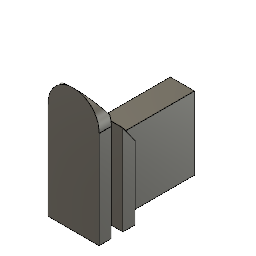
1010RailButton (Autodesk Fusion 360 design; units mm, degrees)
Autodesk Fusion 360 part; units mm, degrees
note: some values were not read from the file. Set by a fixed rule: which sketch regions a step uses.
sketch "Sketch1" plane through (0, 0, 0) normal (0, 0, 1) x (1, 0, 0)
  circle A0 centre (0, 0) radius 5.25
  dimension "d1" = 10.5
  constraint coincident A0.centre origin
  measures "d1" diameter of A0
extrude "Extrude1" add sketch "Sketch1" along normal blind 2.5 makes body 1
sketch "Sketch2" plane through (0, 0, 2.5) normal (0, 0, 1) x (1, 0, 0)
  circle A0 centre (0, 0) radius 5.25
  circle A1 centre (0, 0) radius 2.75
  dimension "d4" = 5.5
  constraint concentric A0 A1
  measures "d4" diameter of A1
extrude "Extrude2" add sketch "Sketch2" along normal blind 2.4 contours A1 bodies 1
sketch "Sketch3" plane through (0, 0, 4.9) normal (0, 0, 1) x (1, 0, 0)
  circle A0 centre (0, 0) radius 2.75
  circle A1 centre (0, 0) radius 5.25
  dimension "d7" = 10.5
  constraint concentric A0 A1
  measures "d7" diameter of A1
extrude "Extrude3" add sketch "Sketch3" along normal blind 2.5 contours A0 | A1 bodies 1
fillet "Fillet1" radius 0.5 2 edges at (-2.5639, 0.9944, 2.5) (-2.5639, -0.9944, 4.9) on bodies 1
sketch "Sketch4" plane through (0, 0, 0) normal (0, 0, -1) x (-1, 0, 0)
  circle A0 centre (0, 0) radius 5.25
  circle A1 centre (0, 0) radius 2.75
  dimension "d11" = 5.5
  constraint concentric A0 A1
  measures "d11" diameter of A1
extrude "Extrude4" add sketch "Sketch4" along normal blind 10 contours A1 bodies 1
fillet "Fillet2" radius 0.5 1 edges at (2.5639, 0.9944, 0) on bodies 1
delete_body "RemoveBody1" bodies 1
sketch "Sketch5" plane through (0, 0, 0) normal (0, 1, 0) x (1, 0, 0)
sketch "Sketch6" plane through (0, 0, 0) normal (0, 0, 1) x (1, 0, 0)
  line L0 (0, 0) -> (5.25, 0)
  line L1 (0, 0) -> (-5.25, 0)
  line L2 (5.25, 0) -> (5.25, 15)
  line L3 (5.25, 15) -> (-5.25, 15)
  line L4 (-5.25, 15) -> (-5.25, 0)
  circle A0 centre (0, 15) radius 5.25
  dimension "d15" = 5.25
  dimension "d16" = 5.25
  dimension "d17" = 15
  dimension "d18" = 10.5
  constraint coincident L0.start L1.start
  constraint horizontal L0
  constraint parallel L0 L1
  constraint perpendicular L0 L2
  constraint perpendicular L2 L3
  constraint perpendicular L1 L4
  constraint midpoint L3 A0.centre
  measures "d15" distance of L0.start L0.end
  measures "d16" distance of L0.start L1.end
  measures "d17" distance of L0.end L2.end
  measures "d18" diameter of A0
extrude "Extrude5" add sketch "Sketch6" along normal blind 2.5 separate body makes body 2
sketch "Sketch7" plane through (0, 0, 2.5) normal (0, 0, 1) x (1, 0, 0)
  line L0 (-5.25, 0) -> (5.25, 0)
  line L1 (5.25, 0) -> (5.25, 15)
  arc A0 (5.25, 15) -> (-5.25, 15) centre (0, 15) ccw
  line L2 (-5.25, 15) -> (-5.25, 0)
  line L3 (0, 0) -> (2.75, 0)
  line L4 (0, 0) -> (-2.75, 0)
  line L5 (-2.75, 0) -> (-2.75, 12.5)
  line L6 (2.75, 0) -> (2.75, 12.5)
  line L7 (2.75, 12.5) -> (-2.75, 12.5)
  circle A1 centre (0, 12.5) radius 2.75
  dimension "d21" = 2.75
  dimension "d22" = 2.75
  dimension "d23" = 12.5
  dimension "d24" = 5.5
  constraint coincident L3.start L4.start
  constraint coincident L0 L3.end
  constraint parallel L0 L4
  constraint perpendicular L0 L5
  constraint perpendicular L0 L6
  constraint perpendicular L5 L7
  constraint midpoint L7 A1.centre
  measures "d21" distance of L3.start L3.end
  measures "d22" distance of L3.start L4.end
  measures "d23" distance of L4.end L5.end
  measures "d24" diameter of A1
extrude "Extrude6" add sketch "Sketch7" along normal blind 2.4 contours L0 L3 L4 L5 L6 A1 | L7 A1 | L7 A1 bodies 2
sketch "Sketch8" plane through (0, 0, 4.9) normal (0, 0, 1) x (1, 0, 0)
  line L0 (-2.75, 0) -> (2.75, 0)
  line L1 (2.75, 0) -> (2.75, 12.5)
  arc A0 (2.75, 12.5) -> (-2.75, 12.5) centre (0, 12.5) ccw
  line L2 (-2.75, 12.5) -> (-2.75, 0)
  circle A1 centre (0, 15.25) radius 5.25
  line L3 (0, 0) -> (5.25, 0)
  line L4 (5.25, 0) -> (5.25, 15)
  line L5 (0, 0) -> (-5.25, 0)
  line L6 (-5.25, 0) -> (-5.25, 15.25)
  line L7 (5.25, 15) -> (-5.25, 15)
  dimension "d27" = 10.5
  dimension "d39" = 5.25
  dimension "d40" = 15
  dimension "d41" = 5.25
  dimension "d42" = 10.5
  constraint midpoint A0 A1.centre
  constraint coincident L3.start L5.start
  constraint parallel L0 L3
  constraint perpendicular L3 L4
  constraint perpendicular L4 L5
  constraint coincident A1 L6.end
  constraint tangent A1 L6
  constraint perpendicular L4 L7
  measures "d27" diameter of A1
  measures "d39" distance of L3.start L3.end
  measures "d40" distance of L3.end L4.end
  measures "d41" distance of L3.start L5.end
  measures "d42" distance of L4.end L7.end
extrude "Extrude10" add sketch "Sketch8" along normal blind 2.5 contours L0 L1 L2 A1 L3 L5 | L2 A1 L5 L6 L7 | A0 L2 A1 L7 | L1 A0 L2 A1 L7 | L1 A1 L3 L4 L7 | A0 A1 L7 | L1 A0 A1 L7 | A0 L7 bodies 2
extrude "Extrude7" add sketch "Sketch8" along normal blind 2.5 contours L0 L1 L2 A1 L3 L5 | L2 A1 L5 L6 | A0 L2 A1 L7 | L1 A0 L2 A1 L7 | A0 A1 L6 L7 | L1 A0 A1 L7 | A0 L7 bodies 2
sketch "Sketch9" plane through (0, 0, 7.4) normal (0, 0, 1) x (1, 0, 0)
  arc A0 (5.244, 15) -> (-5.244, 15) centre (0, 15.25) ccw
  line L0 (-5.25, 0) -> (5.25, 0)
  line L1 (0, 0) -> (2.5, 0)
  line L2 (0, 0) -> (-2.5, 0)
  line L3 (2.5, 0) -> (2.5, 15)
  line L4 (-2.5, 0) -> (-2.5, 15)
  line L5 (-2.5, 15) -> (2.5, 15)
  line L6 (5.25, 0) -> (5.25, 15)
  line L7 (5.25, 15) -> (5.244, 15)
  line L8 (-5.244, 15) -> (-5.25, 15)
  line L9 (-5.25, 15) -> (-5.25, 0)
  dimension "d30" = 2.5
  dimension "d31" = 2.5
  dimension "d32" = 15
  constraint coincident L1.start L2.start
  constraint parallel L0 L1
  constraint parallel L0 L2
  constraint perpendicular L0 L3
  constraint perpendicular L2 L4
  constraint perpendicular L3 L5
  measures "d30" distance of L1.start L1.end
  measures "d31" distance of L1.start L2.end
  measures "d32" distance of L1.end L3.end
sketch "Sketch11" plane through (0, 0, 0) normal (0, 0, -1) x (-1, 0, 0)
  line L0 (-5.25, 0) -> (5.25, 0)
  line L1 (5.25, 0) -> (5.25, 15)
  arc A0 (5.25, 15) -> (-5.25, 15) centre (0, 15) ccw
  line L2 (-5.25, 15) -> (-5.25, 0)
  line L3 (0, 0) -> (2.5, 0)
  line L4 (0, 0) -> (-2.5, 0)
  line L5 (2.5, 0) -> (2.5, 15)
  line L6 (-2.5, 0) -> (-2.5, 15)
  line L7 (-2.5, 15) -> (2.5, 15)
  dimension "d45" = 2.5
  dimension "d46" = 2.5
  dimension "d47" = 15
  dimension "d48" = 15
  constraint coincident L3.start L4.start
  constraint parallel L0 L3
  constraint parallel L0 L4
  constraint perpendicular L0 L5
  constraint perpendicular L4 L6
  measures "d45" distance of L3.start L3.end
  measures "d46" distance of L3.start L4.end
  measures "d47" distance of L3.end L5.end
  measures "d48" distance of L4.end L6.end
extrude "Extrude11" add sketch "Sketch11" along normal blind 15 contours L0 L3 L4 L5 L6 L7 bodies 2
move_face "OffsetFaces3" offset 5 1 faces at (0.8333, 0, -10) on bodies 2
move_face "OffsetFaces4" offset -5 1 faces at (0.8333, 15, -5) on bodies 2
sketch "Sketch12" plane through (-5.25, 0, 0) normal (-1, 0, 0) x (0, 0, 1)
  line L0 (0, 15) -> (0, -5)
  line L1 (0, -5) -> (2.5, -5)
  line L2 (2.5, -5) -> (2.5, 15)
  line L3 (2.5, 15) -> (0, 15)
  line L4 (0, 10) -> (7.4, 20.5)
  line L5 (7.4, 20.5) -> (1.8481, 24.4128)
  line L6 (1.8481, 24.4128) -> (-5.5519, 13.9128)
  line L7 (-5.5519, 13.9128) -> (0, 10)
  constraint perpendicular L4 L5
  constraint parallel L4 L6
  constraint parallel L5 L7
  constraint coincident L0 L4.start
extrude "Extrude12" cut sketch "Sketch12" against normal up to surface (10.5 mm away) contours L0 L2 L3 L4 | L0 L2 L3 L4 L5 L6 L7 bodies 2
